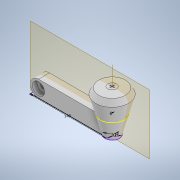
# Autodesk Inventor part: handle
Saved by Autodesk Inventor 2021 (Build 250183000, 183)
## iProperties
Created: 2021-03-11
Part Number: handle
Material: Generic
Document SubType Name: Modeling
Designer: ben
Density: 1 g/cm^3
Appearance: Default
Author: ben
Autodesk Inventor part; units mm, degrees
ref_plane "YZ Plane" through (0, 0, 0) normal (1, 0, 0) x (0, 1, 0)
ref_plane "XZ Plane" through (0, 0, 0) normal (0, 1, 0) x (-1, 0, 0)
ref_plane "XY Plane" through (0, 0, 0) normal (0, 0, 1) x (1, 0, 0)
sketch "Sketch1" plane through (0, 0, 0) normal (0, 0, 1) x (1, 0, 0)
  line L0 (5, -10) -> (-135, -10)
  line L1 (-135, -10) -> (-135, 10)
  line L2 (-135, 10) -> (5, 10)
  line L3 (5, 10) -> (5, -10)
  circle A0 centre (-135, 0) radius 13
  point P0 (0, 0)
  dimension "d0" = 140
  dimension "d1" = 20
  dimension "d5" = 26
  constraints: 8 end point, 2 parallel, 1 centre point, 1 horizontal, 1 horizontal alignment, 1 midpoint, 1 perpendicular
  measures "d0" distance of L1.end L2.end
  measures "d1" distance of L0.end L1.end
  measures "d5" diameter of A0
extrude "Extrusion1" add sketch "Sketch1" along normal blind 30 contours L0 A0 L2 L3 | L0 L1 L2 A0 picked at (-130.6667, 0)
fillet "Fillet1" radius 15 2 edges at (5, 0, 30) (5, 0, 0)
sketch "Sketch9" plane through (-10, 10, 15) normal (0, 1, 0) x (1, 0, 0)
  circle A0 centre (0, 0) radius 11.2
  point P0 (10, 15)
  dimension "d21" = 22.4
  constraints: 1 centre point
  measures "d21" diameter of A0
extrude "Extrusion8" cut sketch "Sketch9" against normal through all
ref_plane "Work Plane4" through (-10, 0, 15) normal (0, 1, 0) x (1, 0, 0)
sketch "Sketch19" plane through (-10, 0, 15) normal (0, 1, 0) x (1, 0, 0)
  circle A0 centre (0, 0) radius 11.2 projected
  circle A1 centre (0, 0) radius 4
  point P0 (10, 15)
  dimension "d59" = 8
  constraints: 1 centre point, 1 coincident
  measures "d59" diameter of A1
extrude "Extrusion19" add sketch "Sketch19" along normal mid plane 4
sketch "Sketch23" plane through (-10, 0, 15) normal (0, 1, 0) x (1, 0, 0)
  line L0 (-103, -19) -> (-94.9615, -49)
  line L1 (-94.9615, -49) -> (-100.735, -59)
  line L2 (-103, -19) -> (-113.8, -19)
  line L3 (-125, -15) -> (0, -15) projected
  line L4 (-113.8, -19) -> (-113.8, -26.4)
  line L5 (-113.8, -26.4) -> (-121, -26.4)
  line L6 (-125, -76.2) -> (-125, 30.2) projected
  line L7 (-117, -59) -> (-117, -61)
  line L8 (-119, -59) -> (-119, -51)
  line L9 (-119, -59) -> (-111, -59) construction
  line L10 (-119, -51) -> (-121, -51)
  line L11 (-117, -61) -> (-100.735, -59)
  line L12 (-121, -51) -> (-121, -26.4)
  line L13 (-117, -59) -> (-119, -59)
  point P0 (10, 15)
  point P1 (-125, -19)
  dimension "d64" = 75
  dimension "d65" = 30
  dimension "d66" = 10
  dimension "d67" = 135
  dimension "d70" = 7.4
  dimension "d72" = 7.2
  dimension "d75" = 2
  dimension "d76" = 8
  dimension "d82" = 11.2
  dimension "d98" = 4
  dimension "d113" = 4
  dimension "d114" = 22
  constraints: 24 end point, 3 horizontal, 3 vertical, 2 perpendicular, 1 point on line, 1 other
  measures "d64" angle to the sketch x axis of L0
  measures "d65" vertical distance of L0.start L0.end
  measures "d66" vertical distance of L1.end L0.end
  measures "d67" angle of L0 L1
  measures "d70" distance of L2.end L4.end
  measures "d72" distance of L4.end L5.end
  measures "d75" distance of L7.start L7.end
  measures "d76" distance of L8.start L8.end
  measures "d82" distance between parallel lines of L6 L4
  measures "d114" distance from line of L6 L0.start
sketch "Sketch26" plane through (-10, 0, 15) normal (0, 1, 0) x (1, 0, 0)
  line L0 (-138, 15) -> (-112, 15) projected
  line L1 (-125, 15) -> (-112, 15)
  line L2 (-125, -25.8) -> (-125, 21.8) projected
  line L3 (-125, 15) -> (0, 15) projected
  line L4 (-102.8897, -19) -> (-125, -19)
  line L5 (-125, -19) -> (-125, 15)
  line L6 (-112, 15) -> (-102.8897, -19)
  point P0 (10, 15)
  point P1 (-125, -15)
  dimension "d111" = 4
  dimension "d112" = 75
  constraints: 8 end point, 2 perpendicular, 1 collinear, 1 point on line
  measures "d111" distance of point (-125, -15) L4.end
  measures "d112" angle of L3 L6
revolve "Revolution2" add sketch "Sketch26" angle 360 about axis through (-135, 0, 30) along (0, 0, -1)
sketch "Sketch27" plane through (-135, 0, 34) normal (0, 0, 1) x (0, -1, 0)
  circle A0 centre (0, 0) radius 4
  circle A1 centre (0, 0) radius 22.1103 projected
  dimension "d79" = 8
  constraints: 1 centre point
  measures "d79" diameter of A0
extrude "Extrusion21" add sketch "Sketch27" along normal blind 32 contours A0
revolve "Revolution3" add sketch "Sketch23" angle 360 about axis through (-135, 0, 30) along (0, 0, -1) separate body
sketch "Sketch28" plane through (-10, 0, 15) normal (0, 1, 0) x (1, 0, 0)
  line L0 (-133, -61) -> (-117, -61) projected
  line L1 (-133, -59) -> (-117, -59) projected
  line L2 (-131, -59) -> (-119, -59) projected
  line L3 (-131, -51) -> (-119, -51) projected
  line L4 (-117, -61) -> (-117, -59) projected
  line L5 (-133, -61) -> (-133, -59) projected
  line L6 (-131, -59) -> (-131, -51) projected
  line L7 (-119, -59) -> (-119, -51) projected
  line L8 (-125, -76.2) -> (-125, 30.2) projected
  point P0 (10, 15)
  point P1 (-125, -51)
  point P2 (-125, -61)
revolve "Revolution4" add sketch "Sketch28" angle 360 about axis through (-135, 0, 30) along (0, 0, -1) separate body contours L8 L1 L4 L0 | L8 L3 L7 L1
sketch "Sketch29" plane through (-135, 0, 76) normal (0, 0, 1) x (1, 0, 0)
  line L0 (4, -0.5) -> (-4, -0.5)
  line L1 (-4, -0.5) -> (-4, 0.5)
  line L2 (-4, 0.5) -> (4, 0.5)
  line L3 (4, 0.5) -> (4, -0.5)
  line L4 (4, -0.5) -> (-4, 0.5) construction
  line L5 (-4, -0.5) -> (4, 0.5) construction
  line L6 (0.5, 4) -> (-0.5, 4)
  line L7 (-0.5, 4) -> (-0.5, -4)
  line L8 (-0.5, -4) -> (0.5, -4)
  line L9 (0.5, -4) -> (0.5, 4)
  line L10 (0.5, 4) -> (-0.5, -4) construction
  line L11 (-0.5, 4) -> (0.5, -4) construction
  point P0 (135, 0)
  point P1 (0, 0)
  point P2 (0, 0)
  point P3 (0, 0)
  point P4 (0, 0)
  point P5 (0, 0)
  point P6 (0, 0)
  point P7 (0.5, 0.5)
  point P8 (-0.5, 0.5)
  point P9 (-0.5, -0.5)
  point P10 (0.5, -0.5)
  dimension "d92" = 8
  dimension "d93" = 1
  dimension "d94" = 1
  dimension "d95" = 8
  constraints: 24 end point, 7 midpoint, 4 parallel, 2 coincident, 2 horizontal, 2 perpendicular
  measures "d92" distance of L1.end L2.end
  measures "d93" distance of L0.end L1.end
  measures "d94" distance of L8.end L7.end
  measures "d95" distance of L7.end L6.end
extrude "Extrusion22" cut sketch "Sketch29" against normal blind 2 bodies 3
thicken "Thicken1" [suppressed]
thicken "Thicken2" [suppressed]
thicken "Thicken3" [suppressed]
thicken "Thicken4" [suppressed]
thicken "Thicken5" [suppressed]
sketch "Sketch30" plane through (-135, 0, 66) normal (0, 0, 1) x (1, 0, 0)
  circle A0 centre (0, 0) radius 2
  dimension "d115" = 4
  constraints: 1 centre point
  measures "d115" diameter of A0
extrude "Extrusion23" cut sketch "Sketch30" against normal blind 10 bodies 1
thread "Thread3" size "M4x0.5" class "6H" standard "ANSI Metric M Profile" full length
sketch "Sketch31" plane through (-135, 0, 66) normal (0, 0, -1) x (-1, 0, 0)
  circle A0 centre (0, 0) radius 2
  dimension "d120" = 4
  constraints: 1 centre point
  measures "d120" diameter of A0
extrude "Extrusion24" add sketch "Sketch31" along normal blind 10 bodies 3
thread "Thread4" size "M4x0.5" class "6g" standard "ANSI Metric M Profile" full length
